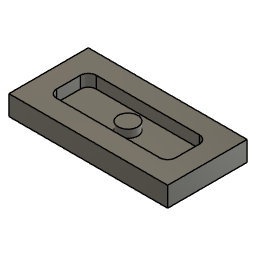
First nc code v1 (Autodesk Fusion 360 design; units mm, degrees)
Autodesk Fusion 360 part; units mm, degrees
sketch "Sketch1" plane through (0, 0, 0) normal (0, 1, 0) x (1, 0, 0)
  line L0 (100, -50) -> (-100, -50)
  line L1 (-100, -50) -> (-100, 50)
  line L2 (-100, 50) -> (100, 50)
  line L3 (100, 50) -> (100, -50)
  line L4 (100, -50) -> (-100, 50) construction
  line L5 (-100, -50) -> (100, 50) construction
  line L6 (65, -25) -> (-65, -25)
  line L7 (-75, -15) -> (-75, 15)
  line L8 (-65, 25) -> (65, 25)
  line L9 (75, 15) -> (75, -15)
  line L10 (75, -25) -> (-75, 25) construction
  line L11 (-75, -25) -> (75, 25) construction
  circle A0 centre (0, 0) radius 12.5
  arc A1 (-65, 25) -> (-75, 15) centre (-65, 15) ccw
  arc A2 (-75, -15) -> (-65, -25) centre (-65, -15) ccw
  arc A3 (65, -25) -> (75, -15) centre (65, -15) ccw
  arc A4 (75, 15) -> (65, 25) centre (65, 15) ccw
  dimension "d1" = 200
  dimension "d2" = 100
  dimension "d3" = 150
  dimension "d4" = 50
  dimension "d5" = 25
  dimension "d6" = 10
  constraint horizontal L0
  constraint perpendicular L0 L1
  constraint parallel L0 L2
  constraint parallel L1 L3
  constraint coincident L4 A0.centre
  constraint coincident L5 A0.centre
  constraint coincident A0.centre origin
  constraint horizontal L6
  constraint perpendicular L6 L7
  constraint parallel L6 L8
  constraint parallel L7 L9
  constraint coincident L10 A0.centre
  constraint coincident L11 A0.centre
  constraint coincident L10.end L8
  constraint coincident L10.end L7
  constraint tangent L8 A1
  constraint tangent L7 A1
  constraint coincident L11.start L7
  constraint coincident L11.start L6
  constraint tangent L7 A2
  constraint tangent L6 A2
  constraint equal A1 A2
  constraint coincident L10.start L6
  constraint coincident L10.start L9
  constraint tangent L6 A3
  constraint tangent L9 A3
  constraint equal A1 A3
  constraint coincident L11.end L9
  constraint coincident L11.end L8
  constraint tangent L9 A4
  constraint tangent L8 A4
  constraint equal A1 A4
  measures "d1" distance of L1.end L2.end
  measures "d2" distance of L0.end L1.end
  measures "d3" distance of L10.end L11.end
  measures "d4" distance of L11.start L10.end
  measures "d5" diameter of A0
  measures "d6" radius of A1
extrude "Extrude1" add sketch "Sketch1" along normal blind 25 contours L0 L1 L2 L3
extrude "Extrude2" add sketch "Sketch1" along normal blind 10 contours L6 L7 L8 L9 A1 A2 A3 A4
extrude "Extrude3" add sketch "Sketch1" along normal blind 20 contours A0
